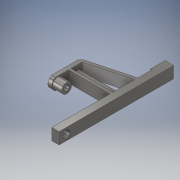
# Autodesk Inventor part: steeringBracket
Saved by Autodesk Inventor 2018 (Build 220112000, 112)
## iProperties
Created: 2018-02-22
Part Number: steeringBracket
Material: Steel, Carbon
Document SubType Name: Modeling
Designer: rochee19
Density: 7.85 g/cm^3
Appearance: Semi-Polished
Mass: 643.155 g
Surface Area: 284.311 cm^2
Volume: 81.9305 cm^3
Author: rochee19
Autodesk Inventor part; units mm, degrees
ref_plane "YZ Plane" through (0, 0, 0) normal (1, 0, 0) x (0, 1, 0)
ref_plane "XZ Plane" through (0, 0, 0) normal (0, 1, 0) x (-1, 0, 0)
ref_plane "XY Plane" through (0, 0, 0) normal (0, 0, 1) x (1, 0, 0)
sketch "Sketch1" plane through (0, 0, 0) normal (0, 1, 0) x (-1, 0, 0)
  line L0 (0, 0) -> (12.7, 0)
  line L1 (12.7, 0) -> (12.7, -177.8)
  line L2 (12.7, -177.8) -> (0, -177.8)
  line L3 (0, -177.8) -> (0, 0)
  dimension "d0" = 12.7
  dimension "d1" = 177.8
  constraints: 8 end point, 2 parallel, 1 horizontal, 1 perpendicular
  measures "d0" distance of L1.end L2.end
  measures "d1" distance of L0.end L1.end
extrude "Extrusion1" add sketch "Sketch1" along normal blind 20.574
sketch "Sketch4" plane through (0, 0, 0) normal (0, -1, 0) x (1, 0, 0)
  line L0 (0, -177.8) -> (-12.7, -177.8) projected
  line L1 (-12.7, -177.8) -> (0, -177.8)
  line L2 (0, -177.8) -> (0, -146.7612)
  line L3 (0, -146.7612) -> (-12.7, -146.7612)
  line L4 (-12.7, -146.7612) -> (-12.7, -177.8)
  line L5 (-12.7, -146.7612) -> (-86.3035, -127.0392)
  line L6 (-12.7, -146.7612) -> (63.5, -146.7612) construction
  line L7 (-86.3035, -127.0392) -> (-86.3035, -73.6992)
  line L8 (-86.3035, -73.6992) -> (-93.4155, -73.6992)
  line L9 (-93.4155, -73.6992) -> (-93.4155, -127.0392)
  line L10 (-12.7, -177.8) -> (0, -177.8)
  line L11 (0, -177.8) -> (0, -152.4)
  line L12 (0, -152.4) -> (-12.7, -152.4)
  line L13 (-12.7, -152.4) -> (-12.7, -177.8)
  line L14 (-12.7, -152.4) -> (-87.7132, -132.3003)
  line L15 (-87.7132, -132.3003) -> (-93.4155, -127.0392)
  point P0 (0, 0)
  dimension "d6" = 12.7
  dimension "d7" = 31.0388
  dimension "d8" = 76.2
  dimension "d9" = 165
  dimension "d10" = 53.34
  dimension "d11" = 7.112
  dimension "d12" = 12.7
  dimension "d13" = 25.4
  constraints: 30 end point, 5 parallel, 3 horizontal, 3 perpendicular, 1 equal length, 1 vertical
  measures "d6" distance of L3.end L2.end
  measures "d7" distance of L2.end L1.end
  measures "d8" distance of L3.end L5.end
  measures "d9" angle of L6 L5
  measures "d10" distance of L5.end L7.end
  measures "d11" distance of L7.end L8.end
  measures "d12" distance of L12.end L11.end
  measures "d13" distance of L11.end L10.end
sketch "Sketch5" plane through (-12.7, 0, -177.8) normal (-1, 0, 0) x (0, 0, 1)
  line L0 (177.8, 20.574) -> (0, 20.574) projected
  line L1 (0, 0) -> (177.8, 0) projected
  line L2 (0, 20.574) -> (31.0403, 20.574)
  line L3 (31.0403, 20.574) -> (31.0403, 0)
  line L4 (31.0403, 0) -> (0, 0)
  line L5 (0, 0) -> (0, 20.574)
  line L6 (31.0403, 10.287) -> (56.4403, 10.287)
  line L7 (56.4403, 10.287) -> (56.4403, 12.319)
  line L8 (56.4403, 12.319) -> (56.4403, 8.255)
  line L9 (56.4403, 8.255) -> (70.3595, 8.255)
  line L10 (70.3595, 8.255) -> (70.3595, 12.319)
  line L11 (70.3595, 12.319) -> (56.4403, 12.319)
  line L12 (70.3595, 12.319) -> (70.3595, 20.574)
  line L13 (70.3595, 8.255) -> (70.3595, 0)
  line L14 (70.3595, 20.574) -> (74.4235, 20.574)
  line L15 (74.4235, 20.574) -> (74.4235, 0)
  line L16 (70.3595, 0) -> (74.4235, 0)
  dimension "d14" = 25.4
  dimension "d15" = 2.032
  dimension "d16" = 4.064
  dimension "d17" = 13.9192
  dimension "d18" = 4.064
  constraints: 30 end point, 8 point on line, 5 perpendicular, 2 horizontal, 2 parallel, 1 collinear, 1 midpoint, 1 vertical
  measures "d14" distance of L6.start L6.end
  measures "d15" distance of L6.end L7.end
  measures "d16" distance of L7.end L8.end
  measures "d17" distance of L8.end L9.end
  measures "d18" distance of L12.end L14.end
extrude "Extrusion2" add sketch "Sketch5" along normal blind 73.66 contours L15 L1 L13 L10 L12 L0 | L10 L9 L8 L7 L11
extrude "Extrusion3" add sketch "Sketch4" against normal blind 20.32 contours L14 L15 L9 L8 L7 L5 L4
sketch "Sketch6" plane through (-12.7, 0, 0) normal (-1, 0, 0) x (0, 0, 1)
  line L0 (0, 0) -> (0, 20.574) projected
  line L1 (0, 10.287) -> (-6.35, 10.287)
  line L2 (-6.35, 10.287) -> (-19.05, 10.287)
  circle A0 centre (-12.7, 10.287) radius 6.35
  dimension "d24" = 12.7
  dimension "d25" = 12.7
  constraints: 4 end point, 2 horizontal, 2 midpoint, 1 horizontal alignment, 2 other
  measures "d24" distance of L1.end L2.end
  measures "d25" distance from line of L0 point (-12.7, 10.287)
extrude "Extrusion4" cut sketch "Sketch6" against normal blind 20.32
sketch "Sketch7" plane through (0, 20.32, 0) normal (0, 1, 0) x (1, 0, 0)
  line L0 (-86.3035, 73.6992) -> (-86.3035, 103.3765) projected
  line L1 (-93.4155, 73.6992) -> (-86.3035, 73.6992) projected
  line L2 (-86.3035, 73.6992) -> (-93.4155, 73.6992)
  line L3 (-93.4155, 73.6992) -> (-93.4155, 127.0392) projected
  line L4 (-93.4155, 73.6992) -> (-93.4155, 127.0392)
  line L5 (-93.4155, 127.0392) -> (-87.7132, 132.3003) projected
  line L6 (-93.4155, 127.0392) -> (-87.7132, 132.3003)
  line L7 (-12.7, 146.7612) -> (-86.3035, 127.0392) projected
  line L8 (-86.3035, 73.6992) -> (-86.3035, 127.0392)
  line L9 (-86.3035, 127.0392) -> (-12.7, 146.7612)
  line L10 (-12.7, 177.8) -> (-12.7, 107.4405) projected
  line L11 (-12.7, 146.7612) -> (-12.7, 152.4)
  line L12 (-87.7132, 132.3003) -> (-12.7, 152.4) projected
  line L13 (-12.7, 152.4) -> (-87.7132, 132.3003)
  point P0 (0, 0)
  dimension "d30" = 76.2
  dimension "d31" = 5.6388
  constraints: 14 end point, 3 collinear, 2 point on line, 1 perpendicular, 1 vertical
  measures "d30" distance of L7.end L9.end
  measures "d31" distance of L9.end L11.end
extrude "Extrusion5" add sketch "Sketch7" along normal blind 0.254
sketch "Sketch8" plane through (-93.4155, 0, -127.0392) normal (-1, 0, 0) x (0, 0, 1)
  line L0 (53.34, 0) -> (53.34, 20.574) projected
  line L1 (53.34, 20.574) -> (46.736, 20.574)
  line L2 (0, 20.574) -> (53.34, 20.574) projected
  line L3 (46.736, 20.574) -> (46.736, 0)
  line L4 (53.34, 0) -> (0, 0) projected
  arc A0 (46.736, 0) -> (46.736, 20.574) centre (42.026, 10.287) ccw
  point P0 (127.0392, 0)
  dimension "d34" = 6.604
  constraints: 4 end point, 2 point on circle, 2 point on line, 1 centre point, 1 perpendicular
  measures "d34" distance of L0.end L1.end
extrude "Extrusion6" cut sketch "Sketch8" against normal blind 25.4 contours L4 A0 L0 | A0 L1 L0
sketch "Sketch9" plane through (-93.4155, 0, -127.0392) normal (-1, 0, 0) x (0, 0, 1)
  arc A0 (46.736, 0) -> (46.736, 20.574) centre (42.026, 10.287) ccw projected
  line L0 (53.34, 10.287) -> (49.276, 10.287)
  line L1 (49.276, 10.287) -> (37.2618, 10.287)
  circle A1 centre (43.2689, 10.287) radius 6.0071
  point P0 (127.0392, 0)
  dimension "d37" = 4.064
  dimension "d38" = 12.0142
  constraints: 4 end point, 2 horizontal, 1 horizontal alignment, 1 midpoint, 1 point on circle, 2 other
  measures "d37" distance of L0.start L0.end
  measures "d38" distance of L0.end L1.end
extrude "Extrusion7" cut sketch "Sketch9" against normal blind 0.508
sketch "Sketch11" plane through (-92.9075, 10.287, -83.7703) normal (-1, 0, 0) x (0, 0, 1)
  circle A0 centre (0, 0) radius 4.826
  point P0 (83.7703, -10.287)
  dimension "d41" = 9.652
  constraints: 1 centre point
  measures "d41" diameter of A0
extrude "Extrusion8" cut sketch "Sketch11" against normal blind 22.86
sketch "Sketch12" plane through (-86.3035, 0, -103.3765) normal (1, 0, 0) x (0, 0, -1)
  circle A0 centre (-19.6062, 10.287) radius 6.0071 projected
  circle A1 centre (-19.6062, 10.287) radius 8.89
  point P0 (-103.3765, 0)
  dimension "d44" = 17.78
  constraints: 1 centre point, 1 coincident
  measures "d44" diameter of A1
extrude "Extrusion9" add sketch "Sketch12" along normal blind 16.002
sketch "Sketch13" plane through (-86.3035, 10.287, -83.7703) normal (1, 0, 0) x (0, 0, -1)
  circle A0 centre (0, 0) radius 4.826 projected
  circle A1 centre (0, 0) radius 4.826
  circle A2 centre (0, 0) radius 6.0071
  point P0 (-83.7703, -10.287)
  constraints: 2 centre point, 2 coincident
extrude "Extrusion10" add sketch "Sketch13" along normal blind 16.002
sketch "Sketch21" plane through (0, 0, -177.8) normal (0, 0, -1) x (-1, 0, 0)
  line L0 (0, 0) -> (12.7, 0)
  line L1 (12.7, 0) -> (12.7, 20.574)
  line L2 (12.7, 20.574) -> (0, 20.574)
  line L3 (0, 20.574) -> (0, 0)
  constraints: 8 end point, 2 parallel, 1 horizontal, 1 perpendicular
extrude "Extrusion14" add sketch "Sketch21" along normal blind 25.4
sketch "Sketch22" plane through (-12.7, 0, -152.4) normal (-1, 0, 0) x (0, 0, 1)
  line L0 (0, 0) -> (-50.8, 0) projected
  line L1 (0, 20.574) -> (-50.8, 20.574) projected
  line L2 (-50.8, 0) -> (-25.4, 0)
  line L3 (-25.4, 0) -> (-25.4, 20.574)
  line L4 (-25.4, 20.574) -> (-50.8, 20.574)
  line L5 (-50.8, 20.574) -> (-50.8, 0)
  point P0 (152.4, 0)
  constraints: 8 end point, 2 parallel, 1 horizontal, 1 midpoint, 1 perpendicular
extrude "Extrusion15" add sketch "Sketch22" along normal blind 2.54
body "Solid1"
